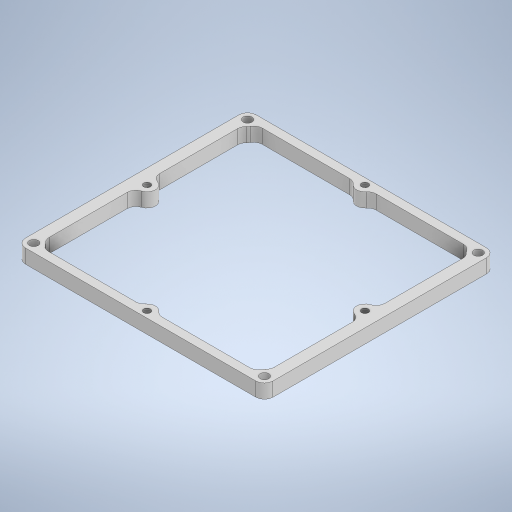
# Autodesk Inventor part: ElectronicsBayMount
Saved by Autodesk Inventor 2023 (Build 270158000, 158)
## iProperties
Created: 2022-08-17
Part Number: ElectronicsBayMount
Material: Generic
Document SubType Name: Modeling
Designer: Aditya Bansal
Density: 1 g/cm^3
Appearance: Default
Author: Aditya Bansal
Autodesk Inventor part; units mm, degrees
ref_plane "YZ Plane" through (0, 0, 0) normal (1, 0, 0) x (0, 1, 0)
ref_plane "XZ Plane" through (0, 0, 0) normal (0, 1, 0) x (-1, 0, 0)
ref_plane "XY Plane" through (0, 0, 0) normal (0, 0, 1) x (1, 0, 0)
sketch "Sketch4" plane through (0, 0, 0) normal (0, 1, 0) x (-1, 0, 0)
  line L0 (0, 0) -> (-88, 0)
  line L1 (-88, 0) -> (-88, -82)
  line L2 (-88, -82) -> (0, -82)
  line L3 (0, -82) -> (0, 0)
  line L4 (-2.25, -82.75) -> (-85.75, -82.75) construction
  line L5 (-85.75, -82.75) -> (-85.75, 0.75) construction
  line L6 (-85.75, 0.75) -> (-2.25, 0.75) construction
  line L7 (-2.25, 0.75) -> (-2.25, -82.75) construction
  circle A0 centre (-44, -79.75) radius 1.6 construction
  circle A1 centre (-82.75, -41) radius 1.6 construction
  circle A2 centre (-5.25, -41) radius 1.6 construction
  circle A3 centre (-44, -2.25) radius 1.6 construction
  arc A4 (-42.0157, -82) -> (-45.9843, -82) centre (-44, -79.75) ccw
  circle A5 centre (-5.25, -41) radius 3
  arc A6 (-45.9843, 0) -> (-42.0157, 0) centre (-44, -2.25) ccw
  circle A7 centre (-82.75, -41) radius 3
  circle A8 centre (-3, -79) radius 1.5 construction
  circle A9 centre (-3, -3) radius 1.5 construction
  circle A10 centre (-85, -3) radius 1.5 construction
  circle A11 centre (-85, -79) radius 1.5 construction
  circle A12 centre (-3, -3) radius 3
  circle A13 centre (-85, -3) radius 3
  circle A14 centre (-85, -79) radius 3
  circle A15 centre (-3, -79) radius 3
  line L8 (-6, -3) -> (-41.0953, -3)
  line L9 (-46.9047, -3) -> (-82, -3)
  line L10 (-84, -76.1716) -> (-84, -43.7272)
  line L11 (-46.9047, -79) -> (-82, -79)
  line L12 (-5.2437, -79) -> (-41.0953, -79)
  line L13 (-4, -76.1716) -> (-4, -43.7272)
  line L14 (-4, -5.8284) -> (-4, -38.2728)
  line L15 (-84, -38.2728) -> (-84, -5.8284)
  point P0 (-3, -82)
  point P1 (0, -79)
  point P2 (0, -3)
  point P3 (-3, 0)
  point P4 (-85, 0)
  point P5 (-88, -3)
  point P6 (-88, -79)
  point P7 (-85, -82)
  point P8 (-6, -79)
  dimension "d40" = 88
  dimension "d41" = 82
  dimension "d42" = 83.5
  dimension "d43" = 2.25
  dimension "d44" = 0.75
  dimension "d45" = 3.2
  dimension "d47" = 3
  dimension "d48" = 3
  dimension "d49" = 3
  dimension "d50" = 3
  dimension "d51" = 41
  dimension "d52" = 44
  dimension "d53" = 6
  dimension "d54" = 3
  dimension "d55" = 3
  dimension "d56" = 3
  dimension "d57" = 3
  dimension "d58" = 3
  dimension "d59" = 6
  dimension "d60" = 3
  dimension "d61" = 3
  dimension "d62" = 4
  dimension "d63" = 4
  constraints: 32 end point, 18 point on circle, 15 centre point, 9 equal radius, 8 coincident, 7 parallel, 6 point on line, 5 vertical alignment, 4 collinear, 3 horizontal, 3 horizontal alignment, 3 perpendicular, 6 other
  measures "d40" distance of L1.end L2.end
  measures "d41" distance of L0.end L1.end
  measures "d42" distance of L4.start L4.end
  measures "d43" distance between parallel lines of L1 L5
  measures "d44" distance between parallel lines of L6 L0
  measures "d45" diameter of A1
  measures "d47" distance from line of A0.centre L4
  measures "d48" distance from line of L6 A3.centre
  measures "d49" distance from line of L7 A2.centre
  measures "d50" distance from line of L5 A1.centre
  measures "d51" distance from line of L2 A2.centre
  measures "d52" distance from line of L1 A3.centre
  measures "d53" diameter of A6
  measures "d54" diameter of A9
  measures "d55" distance from line of L3 A9.centre
  measures "d56" distance from line of L0 A9.centre
  measures "d57" distance from line of L1 A10.centre
  measures "d58" distance from line of L2 A8.centre
  measures "d59" diameter of A12
  measures "d60" distance between parallel lines of L0 L9
  measures "d61" distance between parallel lines of L2 L11
  measures "d62" distance between parallel lines of L3 L14
  measures "d63" distance between parallel lines of L1 L15
extrude "Extrusion2" add sketch "Sketch4" along normal blind 5 contours A6 L0 | L0 A12 L8 A6 | A6 L9 A13 L0 | A12 | A13 | L3 A15 L13 A5 L14 A12 | A13 L15 A7 L10 A14 L1 | A15 | A14 | L2 A4 L12 A15 | A5 | A7 | A14 L11 A4 L2 | L2 A4
sketch "Sketch5" plane through (0, 5, 0) normal (0, 1, 0) x (1, 0, 0)
  arc A0 (84, 43.7272) -> (84, 38.2728) centre (82.75, 41) ccw projected
  arc A1 (41.0953, 79) -> (46.9047, 79) centre (44, 79.75) ccw projected
  arc A2 (46.9047, 3) -> (41.0953, 3) centre (44, 2.25) ccw projected
  arc A3 (4, 38.2728) -> (4, 43.7272) centre (5.25, 41) ccw projected
  point P0 (0, 0)
  constraints: 4 coincident
hole "Hole3" at (44, 5, -79.75) at (82.75, 5, -41) at (44, 5, -2.25) at (5.25, 5, -41) direction (0, -1, 0) diameter 2.459 end through all thread size "M3x0.5" class "6H" standard "ANSI Metric M Profile"
sketch "Sketch6" plane through (0, 5, 0) normal (0, 1, 0) x (1, 0, 0)
  arc A0 (4, 76.1716) -> (6, 79) centre (3, 79) ccw projected
  arc A1 (6, 3) -> (4, 5.8284) centre (3, 3) ccw projected
  arc A2 (82, 79) -> (84, 76.1716) centre (85, 79) ccw projected
  arc A3 (84, 5.8284) -> (82, 3) centre (85, 3) ccw projected
  point P0 (0, 0)
  constraints: 4 coincident
hole "Hole4" at (85, 5, -79) at (85, 5, -3) at (3, 5, -3) at (3, 5, -79) direction (0, -1, 0) diameter 3.2 end through all clearance for "Flat Head Machine Screw" size "M3" standard "Ansi Metric M Profile"
fillet "Fillet2" radius 3 16 edges at (41.0953, 2.5, -79) (46.9047, 2.5, -79) (6, 2.5, -79) (4, 2.5, -76.1716) (4, 2.5, -43.7272) (4, 2.5, -38.2728) (82, 2.5, -79) (84, 2.5, -76.1716) (84, 2.5, -38.2728) (84, 2.5, -43.7272) (82, 2.5, -3) (84, 2.5, -5.8284) (41.0953, 2.5, -3) (46.9047, 2.5, -3) (6, 2.5, -3) (4, 2.5, -5.8284)
equation "\"d43\" = -0.5 * d42 + 0.5 * d40"
equation "\"d44\" = -0.5 * d41 + 0.5 * d42"
equation "\"d48\" = d47"
equation "\"d50\" = d49"
equation "\"d51\" = 0.5 * d41"
equation "\"d52\" = 0.5 * d40"
body "Solid1"
